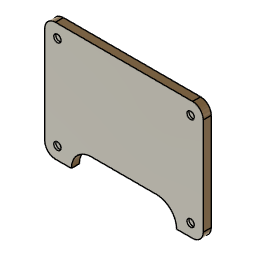
top_access_panel (Autodesk Fusion 360 design; units mm, degrees)
Autodesk Fusion 360 part; units mm, degrees
sketch "Top Access Panel" plane through (0, 0, 0) normal (0, 1, 0) x (1, 0, 0)
  line L0 (0, 0) -> (119, 0)
  line L1 (119, 0) -> (119, -89)
  line L2 (119, -89) -> (0, -89)
  line L3 (0, -89) -> (0, 0)
  dimension "d1" = 119
  dimension "d2" = 89
  constraint horizontal L0
  constraint vertical L1
  constraint horizontal L2
  constraint vertical L3
  constraint coincident L0.start L3.end
  measures "d1" distance of L0.start L0.end
  measures "d2" distance of L0.end L1.end
extrude "Extrude1" add sketch "Top Access Panel" along normal blind 6
fillet "Fillet1" radius 8 4 edges at (0, 3, 89) (119, 3, 89) (119, 3, 0) (0, 3, 0)
sketch "Handle" plane through (0, 6, 0) normal (0, 1, 0) x (-1, 0, 0)
  arc A0 (-8, 0) -> (0, 8) centre (-8, 8) ccw
  line L0 (0, 8) -> (0, 81)
  arc A1 (0, 81) -> (-8, 89) centre (-8, 81) ccw
  line L1 (-8, 89) -> (-111, 89)
  arc A2 (-111, 89) -> (-119, 81) centre (-111, 81) ccw
  line L2 (-119, 81) -> (-119, 8)
  arc A3 (-119, 8) -> (-111, 0) centre (-111, 8) ccw
  line L3 (-111, 0) -> (-8, 0)
  line L4 (-99, 0) -> (-20, 0)
  line L5 (-20, 0) -> (-20, 15)
  line L6 (-20, 15) -> (-99, 15)
  line L7 (-99, 15) -> (-99, 0)
  dimension "d16" = 15
  dimension "d17" = 20
  dimension "d18" = 20
  constraint horizontal L4
  constraint vertical L5
  constraint horizontal L6
  constraint vertical L7
  measures "d16" distance of L4 L6
  measures "d17" distance of L2 L7
  measures "d18" distance of L0 L5
extrude "Extrude3" cut sketch "Handle" against normal blind 6 contours L3 L4 L5 L6 L7
fillet "Fillet2" radius 15 2 edges at (99, 3, 15) (20, 3, 15)
sketch "Sketch4" plane through (0, 0, 0) normal (0, -1, 0) x (1, 0, 0)
  line L0 (35, 15) -> (84, 15)
  arc A0 (99, 0) -> (84, 15) centre (84, 0) ccw
  line L1 (99, 0) -> (111, 0)
  arc A1 (111, 0) -> (119, 8) centre (111, 8) ccw
  line L2 (119, 8) -> (119, 81)
  arc A2 (119, 81) -> (111, 89) centre (111, 81) ccw
  line L3 (111, 89) -> (8, 89)
  arc A3 (8, 89) -> (0, 81) centre (8, 81) ccw
  line L4 (0, 81) -> (0, 8)
  arc A4 (0, 8) -> (8, 0) centre (8, 8) ccw
  line L5 (8, 0) -> (20, 0)
  arc A5 (35, 15) -> (20, 0) centre (35, 0) ccw
  circle A6 centre (9.5, 79.237) radius 2.75
  circle A7 centre (109.5, 79.237) radius 2.75
  circle A8 centre (9.5, 9.237) radius 2.75
  circle A9 centre (109.5, 9.237) radius 2.75
  dimension "d23" = 5.5
  dimension "d24" = 5.5
  dimension "d25" = 5.5
  dimension "d26" = 5.5
  dimension "d27" = 9.5
  dimension "d28" = 9.5
  dimension "d29" = 9.5
  dimension "d30" = 9.5
  dimension "d31" = 9.763
  dimension "d32" = 9.763
  dimension "d33" = 9.237
  dimension "d34" = 9.237
  measures "d23" diameter of A6
  measures "d24" diameter of A7
  measures "d25" diameter of A8
  measures "d26" diameter of A9
  measures "d27" distance of L2 A9.centre
  measures "d28" distance of L4 A8.centre
  measures "d29" distance of L4 A6.centre
  measures "d30" distance of L2 A7.centre
  measures "d31" distance of L3 A6.centre
  measures "d32" distance of L3 A7.centre
  measures "d33" distance of L5 A8.centre
  measures "d34" distance of L1 A9.centre
extrude "Extrude4" cut sketch "Sketch4" against normal blind 1.5 contours A6 | A7 | A8 | A9
equation "mdfThickness = 6 mm" comment "Thickness of the MDF fibre board"
equation "d4 = mdfThickness"
equation "filletRadius = 8 mm" comment "Radius to use for fillets"
equation "d15 = filletRadius"
equation "d19 = -mdfThickness"
equation "d27 = 7.5 mm + ( ( 5.5 / 2 ) * 1 mm ) - 0.25 mm - 0.5 mm"
equation "d28 = 7.5 mm + ( ( 5.5 / 2 ) * 1 mm ) - 0.25 mm - 0.5 mm"
equation "d29 = 7.5 mm + ( ( 5.5 / 2 ) * 1 mm ) - 0.25 mm - 0.5 mm"
equation "d30 = 7.5 mm + ( ( 5.5 / 2 ) * 1 mm ) - 0.25 mm - 0.5 mm"
equation "d31 = 7.763 mm + ( ( 5.5 / 2 ) * 1 mm ) - 0.25 mm - 0.5 mm"
equation "d32 = 7.763 mm + ( ( 5.5 / 2 ) * 1 mm ) - 0.25 mm - 0.5 mm"
equation "d33 = 7.237 mm + ( ( 5.5 / 2 ) * 1 mm ) - 0.25 mm - 0.5 mm"
equation "d34 = 7.237 mm + ( ( 5.5 / 2 ) * 1 mm ) - 0.25 mm - 0.5 mm"
named bodies: "Top Access Panel"
